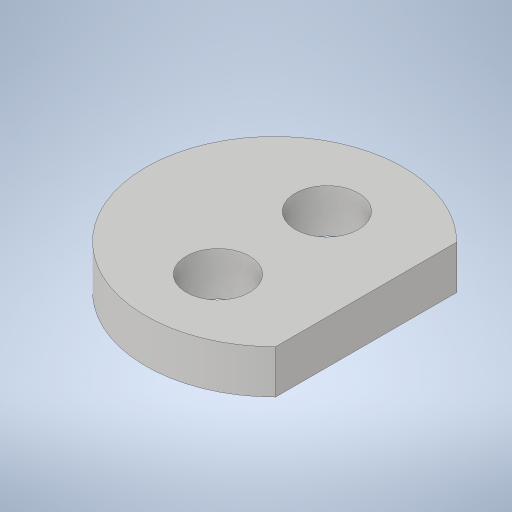
# Autodesk Inventor part: capPRINT4
Saved by Autodesk Inventor 2024.1 (Build 281209000, 209)
## iProperties
Created: 2017-02-09
Part Number: capPRINT4
Material: Generic
Document SubType Name: Modeling
Designer: TDM
Density: 1 g/cm^3
Appearance: Default
Mass: 17.5425 g
Surface Area: 127.561 cm^2
Volume: 17.5425 cm^3
Author: TDM
Autodesk Inventor part; units mm, degrees
ref_plane "YZ Plane" through (0, 0, 0) normal (1, 0, 0) x (0, 1, 0)
ref_plane "XZ Plane" through (0, 0, 0) normal (0, 1, 0) x (-1, 0, 0)
ref_plane "Work Plane5" through (-16.3609, 5.6177, 1.7996) normal (0, 1, 0) x (1, 0, 0)
sketch "Sketch53" plane through (0, 0, 0) normal (0, 1, 0) x (-1, 0, 0)
  circle A0 centre (0, 0) radius 2.953
  line L0 (-2.1, 2.0761) -> (-2.1, -2.0761)
  dimension "d212" = 5.906
  dimension "d213" = 2.1
  constraints: 2 end point, 2 point on circle, 1 centre point, 1 coincident, 1 vertical
  measures "d212" diameter of A0
  measures "d213" distance from line of L0 point (0, 0)
sketch "Sketch54" plane through (0, 0, 0) normal (0, 1, 0) x (-1, 0, 0)
  point P0 (0, 0)
extrude "Extrusion39" add sketch "Sketch53" along normal blind 1 contours A0 L0 picked at (-0.4157, 0)
sketch "Sketch55" plane through (0, 1, 0) normal (0, 1, 0) x (1, 0, 0)
  circle A0 centre (0, -1.2995) radius 0.7245
  circle A1 centre (0, 1.2005) radius 0.7245
  point P0 (0, 0)
  dimension "d218" = 2.5
  constraints: 2 centre point
  measures "d218" distance of A1.centre A0.centre
extrude "Extrusion40" cut sketch "Sketch55" against normal through all
equation "\"PANEL_THICKNESS\" = 3.175"
equation "\"WALL\" = 3"
equation "\"SLACK\" = 1"
body "Solid3"
